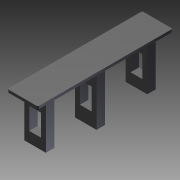
# Autodesk Inventor part: MB2011W01-terminals
Saved by Autodesk Inventor 2015 (Build 190159000, 159)
## iProperties
Category: PARTsolutions
Company: NKKSWITCHES
Created: 2015-01-04
Part Number: MB2011W01-terminals
Catalog Web Link: www.cadenas.de
Description: MB2000 Series - Bushing Mount Miniature Pushbuttons -bm_terminals-
Vendor: NKKSWITCHES
Document SubType Name: Modeling
Designer: PARTuser1
Manufacturer: NKKSWITCHES
Mass: 0.0246775 g
Surface Area: 1.53603 cm^2
Volume: 0.0246775 cm^3
Density: 1 g/cm^3
Material: Generic
Appearance: PSOLRGB-191-191-191
PSOL_IDENT_0: {$CADENAS_DATA\23d-libs\nkkswitches\pushbuttons\mb2000\parts\mb2000_bm_terminals.prj},258 {VTYP=3D},
PSOL_IDENT_1: {NB=MB2011W01-terminals},{LINA=MB2011W01-terminals},{NN=MB2000 Series - Bushing Mount Miniature Push
PSOL_IDENT_2: buttons -bm_terminals},{DATE=21.11.2014 08:56:24},{GEOMDATE=16.01.2009 00:00:00},{VERSION=},{LINEID=
PSOL_IDENT_3: 10},{LINESUBID=-1},{WBVAR=PLSCRCTS,CMR,TRMNLS}  {NB=MB2011W01-terminals},{LINA=MB2011W01-terminals},
PSOL_IDENT_4: {KT=DUMMY},{PN=MB2011W01},{SRS=MB},{PLSCRCTS=2011},{CMR=W},{TRMNLS=01},{A=0},{CMRCLR=0.75,0.75,0.75,
PSOL_IDENT_5: 0.00}
SUPPLIER: NKKSWITCHES
ARTICLENO: MB2011W01-terminals
BOMINFO: MB2011W01-terminals
CREATOR: CADENAS GmbH
Title: MB2011W01-terminals
Author: Cadenas PARTsolutions
Autodesk Inventor part; units mm, degrees
sketch "Sketch_1" plane through (0, 0, 0) normal (0, 1, 0) x (-1, 0, 0)
  line L0 (1.4097, -6.1214) -> (1.4097, 6.1214)
  arc A0 (1.4097, 6.1214) -> (1.2827, 6.2484) centre (1.2827, 6.1214) ccw
  line L1 (1.2827, 6.2484) -> (-1.2827, 6.2484)
  arc A1 (-1.2827, 6.2484) -> (-1.4097, 6.1214) centre (-1.2827, 6.1214) ccw
  line L2 (-1.4097, 6.1214) -> (-1.4097, -6.1214)
  arc A2 (-1.4097, -6.1214) -> (-1.2827, -6.2484) centre (-1.2827, -6.1214) ccw
  line L3 (-1.2827, -6.2484) -> (1.2827, -6.2484)
  arc A3 (1.2827, -6.2484) -> (1.4097, -6.1214) centre (1.2827, -6.1214) ccw
  constraints: 8 end point, 8 point on circle, 4 centre point
extrude "Extrusion1" add sketch "Sketch_1" along normal blind 0.254
sketch "Sketch_2" plane through (0, 0, -4.699) normal (0, 0, 1) x (1, 0, 0)
  line L0 (-1.0033, 0) -> (-1.0033, -4.2418)
  line L1 (-1.0033, -4.2418) -> (1.0033, -4.2418)
  line L2 (1.0033, -4.2418) -> (1.0033, 0)
  line L3 (1.0033, 0) -> (-1.0033, 0)
  line L4 (-0.5461, -1.2446) -> (-0.5461, -3.2512)
  line L5 (-0.5461, -3.2512) -> (0.5461, -3.2512)
  line L6 (0.5461, -3.2512) -> (0.5461, -1.2446)
  line L7 (0.5461, -1.2446) -> (-0.5461, -1.2446)
  constraints: 16 end point
extrude "Extrusion2" add sketch "Sketch_2" along normal mid plane 0.7874
sketch "Sketch_3" plane through (0, 0, 4.699) normal (0, 0, 1) x (1, 0, 0)
  line L0 (-1.0033, 0) -> (-1.0033, -4.2418)
  line L1 (-1.0033, -4.2418) -> (1.0033, -4.2418)
  line L2 (1.0033, -4.2418) -> (1.0033, 0)
  line L3 (1.0033, 0) -> (-1.0033, 0)
  line L4 (-0.5461, -1.2446) -> (-0.5461, -3.2512)
  line L5 (-0.5461, -3.2512) -> (0.5461, -3.2512)
  line L6 (0.5461, -3.2512) -> (0.5461, -1.2446)
  line L7 (0.5461, -1.2446) -> (-0.5461, -1.2446)
  constraints: 16 end point
extrude "Extrusion3" add sketch "Sketch_3" along normal mid plane 0.7874
sketch "Sketch_4" plane through (0, 0, 0) normal (0, 0, 1) x (1, 0, 0)
  line L0 (-1.0033, 0) -> (-1.0033, -4.7498)
  line L1 (-1.0033, -4.7498) -> (1.0033, -4.7498)
  line L2 (1.0033, -4.7498) -> (1.0033, 0)
  line L3 (1.0033, 0) -> (-1.0033, 0)
  line L4 (-0.5461, -1.4986) -> (-0.5461, -3.5052)
  line L5 (-0.5461, -3.5052) -> (0.5461, -3.5052)
  line L6 (0.5461, -3.5052) -> (0.5461, -1.4986)
  line L7 (0.5461, -1.4986) -> (-0.5461, -1.4986)
  constraints: 16 end point
extrude "Extrusion4" add sketch "Sketch_4" along normal mid plane 0.7874
ref_plane "to_body_XY" through (0, 0, 0) normal (0, 1, 0) x (1, 0, 0)
ref_plane "to_body_YZ" through (0, 0, 0) normal (1, 0, 0) x (0, 0, -1)
ref_plane "to_body_ZX" through (0, 0, 0) normal (0, 0, -1) x (0, 1, 0)
body "Solid1"
